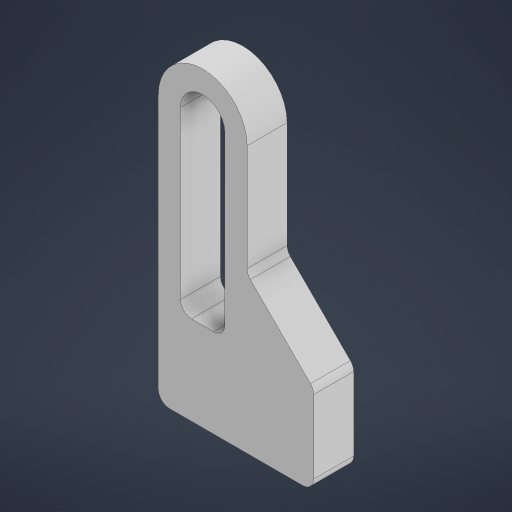
# Autodesk Inventor part: LOCK GUIDE
Saved by Autodesk Inventor 2023 (Build 270158000, 158)
## iProperties
Created: 2024-01-19
Part Number: LOCK GUIDE
Material: Generic
Document SubType Name: Modeling
Designer: User
Density: 1 g/cm^3
Appearance: Default
Author: User
Autodesk Inventor part; units mm, degrees
ref_plane "YZ Plane" through (0, 0, 0) normal (1, 0, 0) x (0, 1, 0)
ref_plane "XZ Plane" through (0, 0, 0) normal (0, 1, 0) x (-1, 0, 0)
ref_plane "XY Plane" through (0, 0, 0) normal (0, 0, 1) x (1, 0, 0)
sketch "Sketch1" plane through (0, 0, 0) normal (0, 0, 1) x (1, 0, 0)
  line L0 (0, 0) -> (70, 0)
  line L1 (70, 0) -> (70, 40)
  line L2 (0, 120) -> (0, 0)
  line L3 (70, 40) -> (40, 70)
  line L4 (40, 120) -> (40, 70)
  line L5 (10, 40) -> (30, 40)
  line L6 (30, 40) -> (30, 120)
  line L7 (10, 120) -> (10, 40)
  arc A0 (40, 120) -> (0, 120) centre (20, 120) ccw
  arc A1 (30, 120) -> (10, 120) centre (20, 120) ccw
  point P0 (20, 40)
  dimension "d8" = 120
  dimension "d13" = 30
  dimension "d15" = 30
  dimension "d16" = 40
  dimension "d17" = 20
  dimension "d20" = 40
  dimension "d21" = 70
  dimension "d22" = 80
  dimension "d23" = 20
  constraints: 16 end point, 4 point on circle, 3 perpendicular, 2 centre point, 2 horizontal, 2 parallel, 1 concentric, 1 horizontal alignment, 1 midpoint
  measures "d8" distance of L2.start L0.start
  measures "d13" distance from line of L3.end L1
  measures "d15" horizontal distance of L1.end L3.end
  measures "d16" distance between parallel lines of L6 L1
  measures "d17" distance of L5.start L5.end
  measures "d20" distance from line of point (20, 40) L0
  measures "d21" distance of L0.start L0.end
  measures "d22" distance of L7.start L5.start
  measures "d23" radius of A0
extrude "Extrusion1" add sketch "Sketch1" along normal blind 18
fillet "Fillet1" radius 5 6 edges at (40, 70, 9) (70, 40, 9) (10, 40, 9) (30, 40, 9) (0, 0, 9) (70, 0, 9)
body "Solid1"
